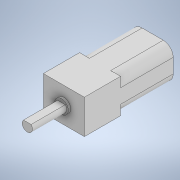
# Autodesk Inventor part: Silniczek
Saved by Autodesk Inventor 2022 (Build 260153000, 153)
## iProperties
Created: 2022-04-03
Part Number: Silniczek
Material: Ogólny
Document SubType Name: Modeling
Designer: jolow
Density: 1 g/cm^3
Appearance: Domyślna
Author: jolow
Autodesk Inventor part; units mm, degrees
ref_plane "YZ Plane" through (0, 0, 0) normal (1, 0, 0) x (0, 1, 0)
ref_plane "XZ Plane" through (0, 0, 0) normal (0, 1, 0) x (-1, 0, 0)
ref_plane "XY Plane" through (0, 0, 0) normal (0, 0, 1) x (1, 0, 0)
sketch "Szkic1" plane through (0, 0, 0) normal (0, 1, 0) x (-1, 0, 0)
  line L0 (0, 0) -> (12, 0)
  line L1 (12, 0) -> (12, 26)
  line L2 (12, 26) -> (0, 26)
  line L3 (0, 26) -> (0, 0)
  dimension "d0" = 26
  dimension "d1" = 12
  constraints: 8 end point, 2 parallel, 1 horizontal, 1 perpendicular
  measures "d0" distance of L0.end L1.end
  measures "d1" distance of L1.end L2.end
extrude "Wyciągnięcie proste1" add sketch "Szkic1" along normal blind 10
fillet "Zaokrąglenie1" radius 2.9 4 edges at (0, 10, 13) (0, 0, 13) (-12, 10, 13) (-12, 0, 13)
sketch "Szkic2" plane through (-9.1, 0, 26) normal (0, 0, 1) x (1, 0, 0)
  circle A0 centre (3.1, 5) radius 2
  line L0 (-2.9, 2.9) -> (-2.9, 7.1) projected
  line L1 (0, 10) -> (6.2, 10) projected
  point P0 (9.1, 0)
  point P1 (-2.9, 5)
  point P2 (3.1, 10)
  dimension "d5" = 4
  constraints: 2 midpoint, 1 centre point, 1 horizontal alignment, 1 vertical alignment
  measures "d5" diameter of A0
extrude "Wyciągnięcie proste2" add sketch "Szkic2" along normal blind 0.7
sketch "Szkic3" plane through (-6, 5, 26.7) normal (0, 0, 1) x (1, 0, 0)
  circle A0 centre (0, 0) radius 1.5
  line L0 (-1.118, 1) -> (1.118, 1)
  circle A1 centre (0, 0) radius 2 projected
  line L1 (-3.1, -5) -> (3.1, -5) projected
  point P0 (6, -5)
  dimension "d8" = 3
  dimension "d9" = 2.5
  dimension "d10" = 0
  dimension "d11" = 0
  constraints: 2 end point, 2 point on circle, 1 centre point, 1 parallel
  measures "d8" diameter of A0
  measures "d10" distance of A1.centre A0.centre
  measures "d11" distance of A1.centre A0.centre
extrude "Wyciągnięcie proste3" add sketch "Szkic3" along normal blind 10 contours A0 L0 picked at (0.0594, 0.1702)
sketch "Szkic4" plane through (0, 10, 0) normal (0, 1, 0) x (1, 0, 0)
  line L0 (-9.1, -26) -> (-12, -26) projected
  line L1 (0, 0) -> (0, -26) projected
  line L2 (-12, -26) -> (0, -26)
  line L3 (0, -26) -> (0, -15.4)
  line L4 (0, -15.4) -> (-12, -15.4)
  line L5 (-12, -15.4) -> (-12, -26)
  line L6 (-2.9, 0) -> (-9.1, 0) projected
  dimension "d14" = 15.4
  constraints: 8 end point, 2 parallel, 1 horizontal, 1 perpendicular, 1 point on line
  measures "d14" distance between parallel lines of L6 L4
extrude "Wyciągnięcie proste4" add sketch "Szkic4" against normal blind 10
